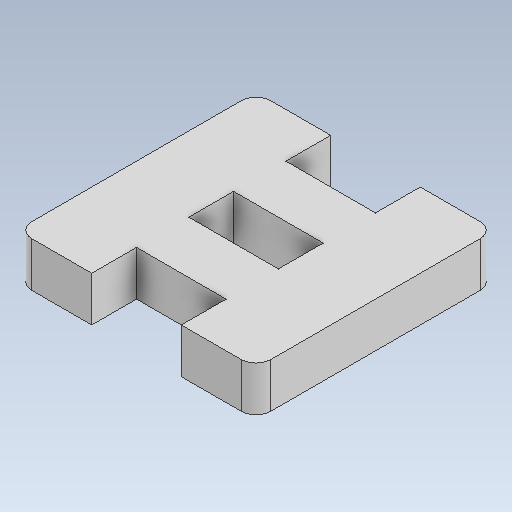
# Autodesk Inventor part: Chwytak wersja 3 - kwadrat_CPY
Saved by Autodesk Inventor 2020 (Build 240168000, 168)
## iProperties
Created: 2019-07-09
Part Number: Chwytak wersja 3 - kwadrat_CPY
Material: Ogólny
Document SubType Name: Modeling
Designer: WIN10
Density: 1 g/cm^3
Appearance: Default
Author: WIN10
Autodesk Inventor part; units mm, degrees
ref_plane "YZ Plane" through (0, 0, 0) normal (1, 0, 0) x (0, 1, 0)
ref_plane "XZ Plane" through (0, 0, 0) normal (0, 1, 0) x (-1, 0, 0)
ref_plane "XY Plane" through (0, 0, 0) normal (0, 0, 1) x (1, 0, 0)
sketch "Szkic1" plane through (0, 0, 0) normal (0, 1, 0) x (-1, 0, 0)
  line L0 (-8, -8) -> (-8, 8)
  line L1 (8, 8) -> (8, -8)
  line L2 (-3, -8) -> (-3, -5)
  line L3 (-3, -5) -> (3, -5)
  line L4 (3, -5) -> (3, -8)
  line L5 (-3, 8) -> (-3, 5)
  line L6 (-3, 5) -> (3, 5)
  line L7 (3, 5) -> (3, 8)
  line L8 (3, 0) -> (3, -1.5)
  line L9 (3, -1.5) -> (-3, -1.5)
  line L10 (-3, -1.5) -> (-3, 1.5)
  line L11 (-3, 1.5) -> (3, 1.5)
  line L12 (3, 1.5) -> (3, 0)
  line L13 (8, -8) -> (3, -8)
  line L14 (-3, -8) -> (-8, -8)
  line L15 (-8, 8) -> (-3, 8)
  line L16 (3, 8) -> (8, 8)
  point P0 (0, 0)
  constraints: 34 end point, 7 parallel, 6 perpendicular, 2 horizontal, 1 point on line, 1 vertical
extrude "Wyciągnięcie proste1" add sketch "Szkic1" along normal mid plane 3
fillet "Zaokrąglenie1" radius 1 4 edges at (-8, 0, -8) (-8, 0, 8) (8, 0, 8) (8, 0, -8)
